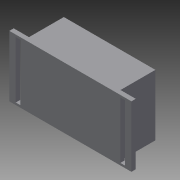
# Autodesk Inventor part: MPB561LaserMount
Saved by Autodesk Inventor 2013 (Build 170138000, 138)
## iProperties
Created: 2014-07-09
Part Number: MPB561LaserMount
Material: Generic
Document SubType Name: Modeling
Designer: 120pa
Density: 1 g/cm^3
Author: 120pa
Autodesk Inventor part; units mm, degrees
ref_plane "YZ Plane" through (0, 0, 0) normal (1, 0, 0) x (0, 1, 0)
ref_plane "XZ Plane" through (0, 0, 0) normal (0, 1, 0) x (-1, 0, 0)
ref_plane "XY Plane" through (0, 0, 0) normal (0, 0, 1) x (1, 0, 0)
sketch "Sketch1" plane through (0, 0, 0) normal (0, 1, 0) x (-1, 0, 0)
  line L0 (0, 0) -> (177.8, 0)
  line L1 (177.8, 0) -> (177.8, 88.9)
  line L2 (177.8, 88.9) -> (0, 88.9)
  line L3 (0, 88.9) -> (0, 0)
  line L4 (9.3218, 3.175) -> (16.0782, 3.175)
  line L5 (16.0782, 3.175) -> (16.0782, 85.725)
  line L6 (16.0782, 85.725) -> (9.3218, 85.725)
  line L7 (9.3218, 85.725) -> (9.3218, 3.175)
  line L8 (9.3218, 3.175) -> (16.0782, 85.725) construction
  line L9 (16.0782, 3.175) -> (9.3218, 85.725) construction
  line L10 (168.4782, 3.175) -> (161.7218, 3.175)
  line L11 (161.7218, 3.175) -> (161.7218, 85.725)
  line L12 (161.7218, 85.725) -> (168.4782, 85.725)
  line L13 (168.4782, 85.725) -> (168.4782, 3.175)
  line L14 (168.4782, 3.175) -> (161.7218, 85.725) construction
  line L15 (161.7218, 3.175) -> (168.4782, 85.725) construction
  point P0 (12.7, 44.45)
  point P1 (165.1, 44.45)
  dimension "d0" = 177.8
  dimension "d1" = 88.9
  dimension "d2" = 6.7564
  dimension "d3" = 82.55
  dimension "d4" = 6.7564
  dimension "d5" = 82.55
  constraints: 32 end point, 4 midpoint
  measures "d0" distance of L2.end L1.end
  measures "d1" distance of L1.end L0.end
  measures "d2" distance of L6.end L5.end
  measures "d3" distance of L5.end L4.end
  measures "d4" distance of L11.end L12.end
  measures "d5" distance of L10.end L11.end
extrude "Extrusion1" add sketch "Sketch1" along normal blind 6.35
sketch "Sketch2" plane through (0, 6.35, 0) normal (0, 1, 0) x (1, 0, 0)
  line L0 (-155.575, 0) -> (-22.225, 0)
  line L1 (-22.225, 0) -> (-22.225, -88.9)
  line L2 (-22.225, -88.9) -> (-155.575, -88.9)
  line L3 (-155.575, -88.9) -> (-155.575, 0)
  line L4 (-155.575, 0) -> (-22.225, -88.9) construction
  line L5 (-22.225, 0) -> (-155.575, -88.9) construction
  point P0 (-88.9, -44.45)
  dimension "d8" = 133.35
  dimension "d9" = 88.9
  constraints: 12 end point, 2 midpoint
  measures "d8" distance of L1.end L2.end
  measures "d9" distance of L0.end L1.end
extrude "Extrusion2" add sketch "Sketch2" along normal blind 50.8
sketch "Sketch3" plane through (0, 57.15, 0) normal (0, 1, 0) x (1, 0, 0)
  line L0 (-149.9, -64.45) -> (-27.9, -64.45)
  line L1 (-27.9, -64.45) -> (-27.9, -24.45)
  line L2 (-27.9, -24.45) -> (-149.9, -24.45)
  line L3 (-149.9, -24.45) -> (-149.9, -64.45)
  line L4 (-149.9, -64.45) -> (-27.9, -24.45) construction
  line L5 (-27.9, -64.45) -> (-149.9, -24.45) construction
  point P0 (0, 0)
  point P1 (-88.9, -44.45)
  dimension "d12" = 122
  dimension "d13" = 40
  constraints: 12 end point, 2 midpoint
  measures "d12" distance of L2.end L1.end
  measures "d13" distance of L1.end L0.end
hole "Hole1" at (-149.9, 57.15, 24.45) at (-149.9, 57.15, 64.45) at (-27.9, 57.15, 24.45) at (-27.9, 57.15, 64.45) direction (0, -1, 0) diameter 2.4638 depth 12.7 tip angle 118
body "Solid1"
